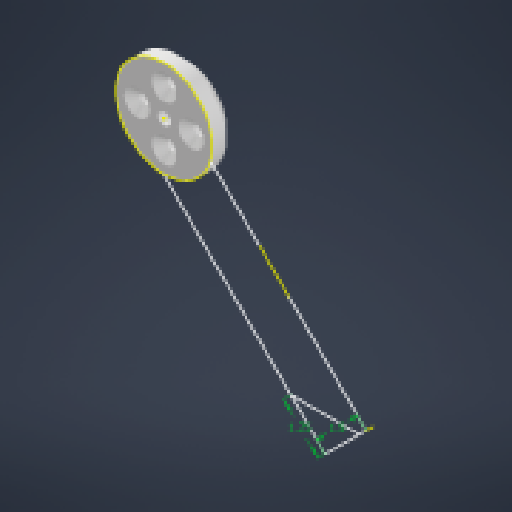
# Autodesk Inventor part: new_custom_servo_claw_bracket
Saved by Autodesk Inventor 2026 (Build 300175000, 175)
## iProperties
Created: 2025-03-29
Part Number: new_custom_servo_claw_bracket
Material: Generic
Document SubType Name: Modeling
Designer: paris
Density: 1 g/cm^3
Appearance: Default
Author: paris
Autodesk Inventor part; units mm, degrees
ref_plane "YZ Plane" through (0, 0, 0) normal (1, 0, 0) x (0, 1, 0)
ref_plane "XZ Plane" through (0, 0, 0) normal (0, 1, 0) x (-1, 0, 0)
ref_plane "XY Plane" through (0, 0, 0) normal (0, 0, 1) x (1, 0, 0)
sketch "Sketch1" plane through (0, 0, 0) normal (0, 0, 1) x (1, 0, 0)
  circle A0 centre (0, 0) radius 9.4
  circle A1 centre (4.949749, 4.949749) radius 1.25
  circle A2 centre (-4.949749, 4.949749) radius 1.25
  circle A3 centre (-4.949749, -4.949749) radius 1.25
  circle A4 centre (0, 0) radius 1.6
  circle A5 centre (4.949749, -4.949749) radius 1.25
  circle A6 centre (0, 0) radius 12.5
  circle A7 centre (0, 0) radius 3.75
  dimension "d0" = 25
  dimension "d31" = 7.5
  constraints: 2 centre point, 2 coincident
  measures "d0" diameter of A6
  measures "d31" diameter of A7
extrude "Extrusion1" add sketch "Sketch1" along normal blind 6 contours A0 | A6 | A7
sketch "Sketch3" plane through (0, 0, 0) normal (0, 1, 0) x (-1, 0, 0)
  line L0 (52.293085, -36.2) -> (52.293085, -39.2)
  line L1 (52.293085, -39.2) -> (35.480704, -39.2)
  line L2 (35.480704, -39.2) -> (35.480704, -35.2)
  line L3 (35.480704, -35.2) -> (51.293085, -35.2)
  line L4 (51.293085, -35.2) -> (52.293085, -36.2)
  line L5 (10.944606, 0.32) -> (11.944606, 1.32) construction
  line L6 (11.944606, 1.32) -> (38.508723, 1.32) construction
  line L7 (38.508723, 1.32) -> (39.508723, 0.32)
  line L8 (39.508723, 0.32) -> (39.508723, -1.18)
  line L9 (39.508723, -1.18) -> (10.944606, -1.18) construction
  line L10 (10.944606, -1.18) -> (10.944606, 0.32) construction
  line L11 (12.5, 0) -> (-12.5, 0)
  line L12 (12.5, 0) -> (10, 0)
  line L13 (12.5, 0) -> (12.5, 2.5)
  line L14 (12.5, 2.5) -> (10, 0)
  line L15 (0, -47.54) -> (0, 10.84)
  point P0 (0, 0)
  dimension "d9" = 2.5
  dimension "d10" = 2.5
  constraints: 28 end point, 4 horizontal, 4 vertical, 1 perpendicular, 1 point on line, 14 other
  measures "d9" distance of L11.start L12.end
  measures "d10" distance of L11.start L13.end
revolve "Revolution2" cut sketch "Sketch3" angle 360 about axis through (0, 0, -10) along (0, 0, 1) contours L11 L14 L13
sketch "Sketch4" plane through (0, 0, 6) normal (0, 0, 1) x (1, 0, 0)
  line L0 (24.631452, -16.169105) -> (32.233463, -23.771115)
  line L1 (24.631452, -16.169105) -> (11.991468, -3.529121)
  circle A0 centre (0, 0) radius 12.5
  line L2 (52.208369, -43.746021) -> (53.976136, -41.978255)
  line L3 (32.233463, -23.771115) -> (52.208369, -43.746021)
  line L4 (52.208369, -43.746021) -> (41.601767, -54.352623)
  line L5 (41.601767, -54.352623) -> (-12.497431, -0.253425)
  line L6 (50.440602, -45.513788) -> (32.762932, -45.513788)
  line L7 (11.991468, -3.529121) -> (10.223701, -1.761354)
  line L8 (10.223701, -1.761354) -> (-0.382901, -12.367955)
  line L9 (-0.382901, -12.367955) -> (-12.497431, -0.253425)
  point P0 (-0.382901, -12.367955)
  dimension "d12" = 15
  dimension "d13" = 12.5
  dimension "d20" = 2.5
  constraints: 16 end point, 3 collinear, 3 perpendicular, 2 point on circle, 2 point on line, 1 horizontal
  measures "d12" distance of L2.start L4.end
  measures "d13" distance of L4.end L6.end
  measures "d20" distance of L1.end L7.end
ref_plane "Work Plane1" through (-4.949749, -4.949749, 0) normal (-0.7071068, 0.7071068, 0) x (0, 0, 1)
extrude "Extrusion2" add sketch "Sketch4" against normal blind 6 contours L0 L3 L4 L6 L5 A0 L1 | A0 L5 L8 L7 picked at (4.096617, -8.795683)
sketch "Sketch5" plane through (-4.949749, -4.949749, 0) normal (-0.7071068, 0.7071068, 0) x (0, 0, 1)
  line L0 (0, -1.25) -> (6, -1.25)
  line L1 (6, -1.25) -> (6, -5.499998)
  line L2 (2.5, 19.500002) -> (6, 19.500002)
  line L3 (0, 17.000002) -> (2.5, 19.500002)
  line L4 (0, -2.999998) -> (0, -1.25)
  line L5 (6, 1.25) -> (0, 1.25)
  line L6 (0, 1.25) -> (0, 5.400002)
  line L7 (0, 5.400002) -> (6, 5.400002)
  line L8 (6, 5.400002) -> (6, 1.25)
  line L9 (6, 15.250004) -> (0, 15.250004)
  line L10 (6, 12.750004) -> (6, 8.600002)
  line L11 (6, 8.600002) -> (0, 8.600002)
  line L12 (0, 8.600002) -> (0, 12.750004)
  line L13 (0, 12.750004) -> (6, 12.750004)
  line L14 (2.5, -5.499998) -> (0, -2.999998)
  line L15 (6, -5.499998) -> (2.5, -5.499998)
  line L16 (6, -1.25) -> (4, -1.25)
  line L17 (6, -1.25) -> (6, -3.25)
  line L18 (6, 19.500002) -> (6, -5.499998)
  line L19 (6, -3.25) -> (4, -1.25)
  line L20 (-1.2, 0) -> (7.2, 0)
  line L21 (6, 19.500002) -> (6, 15.250004)
  line L22 (0, 15.250004) -> (0, 17.000002)
  point P0 (0, 7.000002)
  point P1 (6, -3.25)
  dimension "d14" = 2
  dimension "d15" = 2
  constraints: 6 end point, 1 point on line, 2 other
  measures "d14" distance of L0.end L16.end
  measures "d15" distance of L0.end L17.end
revolve "Revolution3" cut sketch "Sketch5" angle 360 about axis through (-4.949749, -4.949749, 0) along (0, 0, 1) contours L0 L1 L19
pattern_circular "Circular Pattern2" count 4 over 360 about axis through (0, 0, 0) along (0, 0, 1) of "Revolution3"
sketch "Sketch6" plane through (-0.382901, -12.367955, 2.373881) normal (-0.7071068, 0.7071068, 0) x (0.7071068, 0.7071068, 0)
  line L0 (15, 2.373881) -> (15, 1.999565)
  spline S0 degree 2 poles (15, 1.999565) (14.65611, 2.197917) (14.324628, 2.373881) knots 0 0 0 1 1 1 weights 1 1.00054985 1
  line L1 (14.324628, 2.373881) -> (15, 2.373881)
  line L2 (18.204755, -0.126119) -> (18.204755, -3.626119)
  line L3 (18.204755, -3.626119) -> (11.912374, -3.626119)
  line L4 (6.12006, -3.626119) -> (-0.172321, -3.626119)
  line L5 (-0.172321, -3.626119) -> (-0.172321, -0.126119)
  line L6 (0, 0) -> (0, 2.373881)
  line L7 (0, 2.373881) -> (3.707806, 2.373881)
  line L8 (3.707806, 2.373881) -> (14.324628, 2.373881)
  spline S1 degree 2 poles (3.707806, 2.373881) (2.050603, 1.49417) (0, 0) knots 0 0 0 1 1 1 weights 1 1.01402107 1
  point P0 (9.016217, 2.373881)
  constraints: 1 horizontal alignment, 4 other
extrude "Extrusion3" add sketch "Sketch6" along normal up to surface round surface about axis through (0, 0, 1.25) along (0, 0, -1) radius 11.25 half angle -45 far side no
sketch "Sketch7" plane through (50.440602, -45.513788, 0) normal (0.7071068, -0.7071068, 0) x (0.7071068, 0.7071068, 0)
  line L0 (-12.5, 6) -> (0, 6)
  line L1 (-12.5, 6) -> (-12.5, 0)
  line L2 (0, 0) -> (-12.5, 0)
  line L3 (0, 6) -> (0, 0)
  line L4 (0, 6) -> (2.5, 6)
  line L5 (0, 6) -> (0, 0)
  line L6 (2.5, 0) -> (0, 0)
  line L7 (2.5, 6) -> (2.5, 0)
  line L8 (-17.381295, 1.62) -> (-20.312925, 1.62)
  line L9 (-17.381295, 1.62) -> (-12.5, 1.62)
  line L10 (-12.5, 0) -> (-9.5, 0)
  line L11 (-9.5, 0) -> (-9.5, 2)
  line L12 (-9.5, 2) -> (-12.5, 2)
  line L13 (-12.5, 2) -> (-12.5, 0)
  line L14 (-9.5, 2) -> (-7.5, 0)
  line L15 (-9.5, 2) -> (-6.671573, 2) construction
  point P0 (-3.483783, 0)
  point P1 (-12.5, 2)
  dimension "d25" = 3
  dimension "d26" = 2
  dimension "d27" = 45
  constraints: 14 end point, 2 horizontal, 2 parallel, 2 perpendicular, 2 point on line, 1 equal length
  measures "d25" distance of L12.end L11.end
  measures "d26" distance of L11.end L10.end
  measures "d27" angle of L14 L15
extrude "Extrusion4" cut sketch "Sketch7" against normal up to surface contours L12 L11 L2 L1 | L14 L2 L11 round surface about axis through (0, 0, 1.25) along (0, 0, -1) radius 11.25 half angle -45 far side no
sketch "Sketch9" plane through (-4.949749, -4.949749, 0) normal (-0.7071068, 0.7071068, 0) x (0, 0, 1)
  line L0 (6, 17.250004) -> (4, 15.250004)
  line L1 (4, 15.250004) -> (0, 15.250004)
  line L2 (0, 15.250004) -> (0, 17.000002)
  line L3 (0, 17.000002) -> (2.5, 19.500002)
  line L4 (2.5, 19.500002) -> (6, 19.500002)
  line L5 (6, 19.500002) -> (6, 17.250004)
  line L6 (4, 12.750004) -> (6, 10.750004)
  line L7 (6, 10.750004) -> (6, 8.600002)
  line L8 (6, 8.600002) -> (0, 8.600002)
  line L9 (0, 8.600002) -> (0, 12.750004)
  line L10 (0, 12.750004) -> (4, 12.750004)
  line L11 (4, -1.25) -> (6, -3.25)
  line L12 (6, -3.25) -> (6, -5.499998)
  line L13 (6, -5.499998) -> (2.5, -5.499998)
  line L14 (2.5, -5.499998) -> (0, -2.999998)
  line L15 (0, -2.999998) -> (0, -1.25)
  line L16 (0, -1.25) -> (4, -1.25)
  line L17 (6, 3.25) -> (4, 1.25)
  line L18 (4, 1.25) -> (0, 1.25)
  line L19 (0, 1.25) -> (0, 5.400002)
  line L20 (0, 5.400002) -> (6, 5.400002)
  line L21 (6, 5.400002) -> (6, 3.25)
  line L22 (2.5, -5.499998) -> (2.5, 19.500002)
  line L23 (6, 12.983785) -> (2.5, 12.983785)
  line L24 (2.5, 12.983785) -> (2.5, -2.016215)
  line L25 (2.5, -2.016215) -> (6, -2.016215)
  line L26 (6, 12.983785) -> (6, -2.016215)
  line L27 (0, 8.600002) -> (0, 5.400002)
  line L28 (0, 5.400002) -> (0, 8.600002)
  line L29 (0, 7.000002) -> (2.5, 7.000002)
  line L30 (2.5, 7.000002) -> (2.5, 11.000002)
  line L31 (2.5, 11.000002) -> (0, 11.000002)
  line L32 (2.5, 7.000002) -> (2.5, 3.000002)
  line L33 (2.5, 3.000002) -> (0, 2.983785)
  point P0 (2.5, 11.000002)
  dimension "d32" = 2.5
  dimension "d33" = 4
  dimension "d34" = 4
  constraints: 12 end point, 3 perpendicular, 3 point on line
  measures "d32" distance of L29.start L29.end
  measures "d33" distance of L29.end L30.end
  measures "d34" distance of L29.end L32.end
extrude "Extrusion5" cut sketch "Sketch9" along normal blind 25 contours L22 L8 L9 L31 | L22 L29 L27 L8 | L22 L20 L27 L29 | L22 L33 L19 L20
sketch "Sketch10" plane through (-4.949749, -4.949749, 0) normal (-0.7071068, 0.7071068, 0) x (-0.7071068, -0.7071068, 0)
  line L0 (-8.600002, 2.5) -> (-8.600002, 0)
  line L1 (-8.600002, 2.5) -> (-11.000002, 2.5)
  line L2 (-11.000002, 2.5) -> (-11.000002, 0)
  line L3 (-8.600002, 0) -> (-11.000002, 0)
  line L4 (-7.000002, -1.2) -> (-7.000002, 7.2)
  point P0 (-7.000002, 0)
revolve "Revolution4" cut sketch "Sketch10" angle 360 about axis through (0, 0, -10) along (0, 0, 1)
ref_plane "Work Plane2" through (0, 0, -18.75) normal (0, 0, -1) x (-1, 0, 0)
mirror "Mirror1" about plane through (0, 0, -18.75) normal (0, 0, -1) of "Extrusion4", "Extrusion3", "Revolution3", "Circular Pattern2", "Extrusion2", "Revolution2", "Extrusion1"
sketch "Sketch11" plane through (52.208369, -43.746021, 6) normal (0.7071068, 0.7071068, 0) x (0, 0, -1)
  arc A0 (36.443783, 18.378448) -> (35.045362, 17.55589) centre (36.443783, 16.778448) ccw
  arc A1 (33.809543, 17.615975) -> (35.045362, 17.55589) centre (34.442292, 17.891162) ccw
  arc A2 (33.809543, 17.615975) -> (30.083918, 17.860337) centre (31.883783, 16.778448) ccw
  arc A3 (28.824133, 18.044523) -> (30.083918, 17.860337) centre (29.492533, 18.215815) ccw
  arc A4 (28.824133, 18.044523) -> (18.943434, 18.044523) centre (23.883783, 16.778448) ccw
  arc A5 (17.683649, 17.860337) -> (18.943434, 18.044523) centre (18.275033, 18.215815) ccw
  arc A6 (17.683649, 17.860337) -> (13.958024, 17.615975) centre (15.883783, 16.778448) ccw
  arc A7 (12.722205, 17.55589) -> (13.958024, 17.615975) centre (13.325275, 17.891162) ccw
  arc A8 (12.722205, 17.55589) -> (11.323783, 18.378448) centre (11.323783, 16.778448) ccw
  line L0 (11.323783, 22.635) -> (11.323783, 18.378448)
  line L1 (5.71, 28.248783) -> (11.323783, 22.635)
  line L2 (5.71, 38.99965) -> (5.71, 28.248783)
  arc A9 (5.71, 38.99965) -> (6.096638, 39.441716) centre (5.183783, 39.85) ccw
  arc A10 (6.726508, 39.85) -> (6.096638, 39.441716) centre (6.726508, 39.16) ccw
  line L3 (7.800239, 39.85) -> (6.726508, 39.85)
  arc A11 (7.800239, 39.85) -> (8.252787, 40.037452) centre (7.800239, 40.49) ccw
  line L4 (11.21157, 42.996234) -> (8.252787, 40.037452)
  arc A12 (12.296639, 42.446127) -> (11.21157, 42.996234) centre (11.664118, 42.543686) ccw
  arc A13 (12.296639, 42.446127) -> (14.459982, 42.506034) centre (13.383783, 42.278448) ccw
  arc A14 (15.086135, 43.278448) -> (14.459982, 42.506034) centre (15.086135, 42.638448) ccw
  line L5 (15.853783, 43.278448) -> (15.086135, 43.278448)
  arc A15 (16.493783, 42.638448) -> (15.853783, 43.278448) centre (15.853783, 42.638448) ccw
  line L6 (16.493783, 42.638448) -> (16.493783, 27.277734)
  arc A16 (16.493783, 27.277734) -> (18.393783, 25.377734) centre (18.393783, 27.277734) ccw
  line L7 (18.393783, 25.377734) -> (29.373783, 25.377734)
  arc A17 (29.373783, 25.377734) -> (31.273783, 27.277734) centre (29.373783, 27.277734) ccw
  line L8 (31.273783, 27.277734) -> (31.273783, 42.638448)
  arc A18 (31.913783, 43.278448) -> (31.273783, 42.638448) centre (31.913783, 42.638448) ccw
  line L9 (32.681432, 43.278448) -> (31.913783, 43.278448)
  arc A19 (33.307584, 42.506034) -> (32.681432, 43.278448) centre (32.681432, 42.638448) ccw
  arc A20 (33.307584, 42.506034) -> (35.470928, 42.446127) centre (34.383783, 42.278448) ccw
  arc A21 (36.555997, 42.996234) -> (35.470928, 42.446127) centre (36.103449, 42.543686) ccw
  line L10 (39.51478, 40.037452) -> (36.555997, 42.996234)
  arc A22 (39.51478, 40.037452) -> (39.967328, 39.85) centre (39.967328, 40.49) ccw
  line L11 (41.041059, 39.85) -> (39.967328, 39.85)
  arc A23 (41.670929, 39.441716) -> (41.041059, 39.85) centre (41.041059, 39.16) ccw
  arc A24 (41.670929, 39.441716) -> (42.057567, 38.99965) centre (42.583783, 39.85) ccw
  line L12 (42.057567, 28.248783) -> (42.057567, 38.99965)
  line L13 (36.443783, 22.635) -> (42.057567, 28.248783)
  line L14 (36.443783, 18.378448) -> (36.443783, 22.635)
  circle A25 centre (36.443783, 36.16) radius 1.6
  circle A26 centre (11.323783, 36.16) radius 1.6
  circle A27 centre (13.383783, 28.778448) radius 1.1
  circle A28 centre (34.383783, 28.778448) radius 1.1
  arc A29 (35.045362, 16.001006) -> (36.443783, 15.178448) centre (36.443783, 16.778448) ccw
  line L15 (36.443783, 9.11) -> (36.443783, 15.178448)
  line L16 (28.414559, 1.080776) -> (36.443783, 9.11)
  arc A30 (25.805335, 0) -> (28.414559, 1.080776) centre (25.805335, 3.69) ccw
  line L17 (21.962231, 0) -> (25.805335, 0)
  arc A31 (19.353007, 1.080776) -> (21.962231, 0) centre (21.962231, 3.69) ccw
  line L18 (11.323783, 9.11) -> (19.353007, 1.080776)
  line L19 (11.323783, 15.178448) -> (11.323783, 9.11)
  arc A32 (11.323783, 15.178448) -> (12.722205, 16.001006) centre (11.323783, 16.778448) ccw
  arc A33 (13.958024, 15.940921) -> (12.722205, 16.001006) centre (13.325275, 15.665734) ccw
  arc A34 (13.958024, 15.940921) -> (17.683649, 15.696559) centre (15.883783, 16.778448) ccw
  arc A35 (18.943434, 15.512374) -> (17.683649, 15.696559) centre (18.275033, 15.341081) ccw
  arc A36 (18.943434, 15.512374) -> (22.617709, 11.838098) centre (23.883783, 16.778448) ccw
  arc A37 (22.801894, 10.578314) -> (22.617709, 11.838098) centre (22.446417, 11.169698) ccw
  arc A38 (22.801894, 10.578314) -> (24.965672, 10.578314) centre (23.883783, 8.778448) ccw
  arc A39 (25.149858, 11.838098) -> (24.965672, 10.578314) centre (25.32115, 11.169698) ccw
  arc A40 (25.149858, 11.838098) -> (28.824133, 15.512374) centre (23.883783, 16.778448) ccw
  arc A41 (30.083918, 15.696559) -> (28.824133, 15.512374) centre (29.492533, 15.341081) ccw
  arc A42 (30.083918, 15.696559) -> (33.809543, 15.940921) centre (31.883783, 16.778448) ccw
  arc A43 (35.045362, 16.001006) -> (33.809543, 15.940921) centre (34.442292, 15.665734) ccw
  circle A44 centre (23.883783, 3.69) radius 1.6
  line L20 (16.493783, 42.638448) -> (31.273783, 42.638448)
  line L21 (6, 0) -> (6, 59.837863)
  line L22 (43.5, 58.691943) -> (43.5, 7.5)
  line L23 (6, 0) -> (43.5, 0)
  line L24 (43.5, 0) -> (43.5, 45)
  line L25 (43.5, 45) -> (6, 45)
  line L26 (6, 45) -> (6, 0)
  line L27 (13.5, 45) -> (6, 52.5)
  line L28 (13.5, 45) -> (24.106602, 45) construction
  line L29 (36, 45) -> (43.5, 52.5)
  line L30 (36, 45) -> (46.606602, 45) construction
  line L31 (11.323783, 15.178448) -> (11.323783, 18.378448)
  line L32 (36.443783, 18.378448) -> (36.443783, 15.178448)
  line L33 (10.823783, 15.178448) -> (10.823783, 18.378448)
  arc A45 (34.608355, 15.758055) -> (36.443783, 14.678448) centre (36.443783, 16.778448) ccw
  arc A46 (34.608355, 15.758055) -> (34.268057, 15.74151) centre (34.442292, 15.665734) ccw
  arc A47 (29.655378, 15.438967) -> (34.268057, 15.74151) centre (31.883783, 16.778448) ccw
  arc A48 (29.655378, 15.438967) -> (29.308481, 15.388249) centre (29.492533, 15.341081) ccw
  arc A49 (25.273983, 11.35375) -> (29.308481, 15.388249) centre (23.883783, 16.778448) ccw
  arc A50 (25.273983, 11.35375) -> (25.223265, 11.006853) centre (25.32115, 11.169698) ccw
  arc A51 (22.544302, 11.006853) -> (25.223265, 11.006853) centre (23.883783, 8.778448) ccw
  arc A52 (22.544302, 11.006853) -> (22.493584, 11.35375) centre (22.446417, 11.169698) ccw
  arc A53 (18.459086, 15.388249) -> (22.493584, 11.35375) centre (23.883783, 16.778448) ccw
  arc A54 (18.459086, 15.388249) -> (18.112188, 15.438967) centre (18.275033, 15.341081) ccw
  arc A55 (13.49951, 15.74151) -> (18.112188, 15.438967) centre (15.883783, 16.778448) ccw
  arc A56 (13.49951, 15.74151) -> (13.159212, 15.758055) centre (13.325275, 15.665734) ccw
  arc A57 (11.323783, 14.678448) -> (13.159212, 15.758055) centre (11.323783, 16.778448) ccw
  arc A58 (13.159212, 17.798841) -> (11.323783, 18.878448) centre (11.323783, 16.778448) ccw
  arc A59 (13.159212, 17.798841) -> (13.49951, 17.815386) centre (13.325275, 17.891162) ccw
  arc A60 (18.112188, 18.11793) -> (13.49951, 17.815386) centre (15.883783, 16.778448) ccw
  arc A61 (18.112188, 18.11793) -> (18.459086, 18.168648) centre (18.275033, 18.215815) ccw
  arc A62 (29.308481, 18.168648) -> (18.459086, 18.168648) centre (23.883783, 16.778448) ccw
  arc A63 (29.308481, 18.168648) -> (29.655378, 18.11793) centre (29.492533, 18.215815) ccw
  arc A64 (34.268057, 17.815386) -> (29.655378, 18.11793) centre (31.883783, 16.778448) ccw
  arc A65 (34.268057, 17.815386) -> (34.608355, 17.798841) centre (34.442292, 17.891162) ccw
  arc A66 (36.443783, 18.878448) -> (34.608355, 17.798841) centre (36.443783, 16.778448) ccw
  line L34 (36.943783, 18.378448) -> (36.943783, 15.178448)
  circle A67 centre (23.883783, 3.69) radius 2.1
  line L35 (31.773783, 42.638448) -> (31.773783, 27.277734)
  arc A68 (29.373783, 24.877734) -> (31.773783, 27.277734) centre (29.373783, 27.277734) ccw
  line L36 (29.373783, 24.877734) -> (18.393783, 24.877734)
  arc A69 (15.993783, 27.277734) -> (18.393783, 24.877734) centre (18.393783, 27.277734) ccw
  line L37 (15.993783, 27.277734) -> (15.993783, 42.638448)
  line L38 (16.493783, 43.138448) -> (31.273783, 43.138448)
  line L39 (16.493783, 43.138448) -> (15.993783, 42.638448)
  line L40 (31.273783, 43.138448) -> (31.773783, 42.638448)
  line L41 (11.323783, 18.878448) -> (10.823783, 18.378448)
  line L42 (10.823783, 15.178448) -> (11.323783, 14.678448)
  line L43 (36.443783, 18.878448) -> (36.943783, 18.378448)
  line L44 (36.943783, 15.178448) -> (36.443783, 14.678448)
  point P0 (6, 67.85)
  point P1 (25.805335, 0)
  point P2 (6, 45)
  dimension "d38" = 45
  dimension "d39" = 135
  dimension "d40" = 45
  dimension "d41" = 7.5
  dimension "d42" = 7.5
  dimension "d43" = 0.5
  dimension "d44" = 0.5
  dimension "d45" = 0.5
  dimension "d46" = 0.5
  dimension "d47" = 0.5
  dimension "d48" = 0.5
  dimension "d49" = 0.5
  constraints: 48 point on circle, 40 end point, 25 centre point, 6 parallel, 5 perpendicular, 5 point on line, 3 horizontal, 2 equal length, 24 other
  measures "d38" distance of L24.end L23.end
  measures "d39" angle of L28 L27
  measures "d40" angle of L30 L29
  measures "d41" distance of L24.end L29.end
  measures "d42" distance of L25.end L27.end
  measures "d43" distance between parallel lines of L31 L33
  measures "d44" radial gap between concentric circles of A34 A55
  measures "d45" radial gap between concentric circles of A4 A62
  measures "d46" distance between parallel lines of L32 L34
  measures "d47" radial gap between concentric circles of A44 A67
  measures "d48" distance between parallel lines of L7 L36
  measures "d49" distance between parallel lines of L20 L38
extrude "Extrusion6" add sketch "Sketch11" against normal blind 3.5 contours A66 A65 A64 A63 A62 A61 A60 A59 A58 L0 L1 L21 A9 A10 L3 A11 L4 A12 A13 A14 L5 A15 L39 L37 A69 L36 A68 L35 L40 A18 L9 A19 A20 A21 L10 A22 L11 A23 A24 L12 L13 L14 | L14 L13 L12 A24 A23 L11 A22 L10 A21 A20 A19 L9 A18 L40 L38 L39 A15 L5 A14 A13 A12 L4 A11 L3 A10 A9 L21 L25 L22 L24 L23 A30 L16 L15 L44 L34 L43 | L15 L16 A30 L17 A31 L18 L19 A57 A56 A55 A54 A53 A52 A51 A50 A49 A48 A47 A46 A45 | L23 L21 L1 L0 L41 L33 L42 L19 L18 A31 | L25 L29 L22 | L21 L27 L25 | A25 | A26 | A27 | A28
sketch "Sketch12" plane through (49.733495, -46.220895, 6) normal (-0.7071068, -0.7071068, 0) x (0, 0, 1)
  line L0 (-43.5, 0) -> (-6, 0)
  line L1 (-6, 0) -> (-6, 1)
  line L2 (-6, 52.5) -> (-6, 1)
  line L3 (-6, 52.5) -> (-13.5, 45)
  line L4 (-13.5, 45) -> (-36, 45)
  line L5 (-36, 45) -> (-43.5, 52.5)
  line L6 (-43.5, 1) -> (-43.5, 52.5)
  line L7 (-43.5, 1) -> (-43.5, 0)
  line L8 (-31.773783, 42.638448) -> (-31.273783, 43.138448)
  line L9 (-31.273783, 43.138448) -> (-16.493783, 43.138448)
  line L10 (-16.493783, 43.138448) -> (-15.993783, 42.638448)
  line L11 (-15.993783, 42.638448) -> (-15.993783, 27.277734)
  arc A0 (-18.393783, 24.877734) -> (-15.993783, 27.277734) centre (-18.393783, 27.277734) ccw
  line L12 (-18.393783, 24.877734) -> (-29.373783, 24.877734)
  arc A1 (-31.773783, 27.277734) -> (-29.373783, 24.877734) centre (-29.373783, 27.277734) ccw
  line L13 (-31.773783, 27.277734) -> (-31.773783, 42.638448)
  circle A2 centre (-23.883783, 3.69) radius 2.1
  line L14 (-36.943783, 18.378448) -> (-36.443783, 18.878448)
  arc A3 (-34.608355, 17.798841) -> (-36.443783, 18.878448) centre (-36.443783, 16.778448) ccw
  arc A4 (-34.608355, 17.798841) -> (-34.268057, 17.815386) centre (-34.442292, 17.891162) ccw
  arc A5 (-29.655378, 18.11793) -> (-34.268057, 17.815386) centre (-31.883783, 16.778448) ccw
  arc A6 (-29.655378, 18.11793) -> (-29.308481, 18.168648) centre (-29.492533, 18.215815) ccw
  arc A7 (-18.459086, 18.168648) -> (-29.308481, 18.168648) centre (-23.883783, 16.778448) ccw
  arc A8 (-18.459086, 18.168648) -> (-18.112188, 18.11793) centre (-18.275033, 18.215815) ccw
  arc A9 (-13.49951, 17.815386) -> (-18.112188, 18.11793) centre (-15.883783, 16.778448) ccw
  arc A10 (-13.49951, 17.815386) -> (-13.159212, 17.798841) centre (-13.325275, 17.891162) ccw
  arc A11 (-11.323783, 18.878448) -> (-13.159212, 17.798841) centre (-11.323783, 16.778448) ccw
  line L15 (-11.323783, 18.878448) -> (-10.823783, 18.378448)
  line L16 (-10.823783, 18.378448) -> (-10.823783, 15.178448)
  line L17 (-10.823783, 15.178448) -> (-11.323783, 14.678448)
  arc A12 (-13.159212, 15.758055) -> (-11.323783, 14.678448) centre (-11.323783, 16.778448) ccw
  arc A13 (-13.159212, 15.758055) -> (-13.49951, 15.74151) centre (-13.325275, 15.665734) ccw
  arc A14 (-18.112188, 15.438967) -> (-13.49951, 15.74151) centre (-15.883783, 16.778448) ccw
  arc A15 (-18.112188, 15.438967) -> (-18.459086, 15.388249) centre (-18.275033, 15.341081) ccw
  arc A16 (-22.493584, 11.35375) -> (-18.459086, 15.388249) centre (-23.883783, 16.778448) ccw
  arc A17 (-22.493584, 11.35375) -> (-22.544302, 11.006853) centre (-22.446417, 11.169698) ccw
  arc A18 (-25.223265, 11.006853) -> (-22.544302, 11.006853) centre (-23.883783, 8.778448) ccw
  arc A19 (-25.223265, 11.006853) -> (-25.273983, 11.35375) centre (-25.32115, 11.169698) ccw
  arc A20 (-29.308481, 15.388249) -> (-25.273983, 11.35375) centre (-23.883783, 16.778448) ccw
  arc A21 (-29.308481, 15.388249) -> (-29.655378, 15.438967) centre (-29.492533, 15.341081) ccw
  arc A22 (-34.268057, 15.74151) -> (-29.655378, 15.438967) centre (-31.883783, 16.778448) ccw
  arc A23 (-34.268057, 15.74151) -> (-34.608355, 15.758055) centre (-34.442292, 15.665734) ccw
  arc A24 (-36.443783, 14.678448) -> (-34.608355, 15.758055) centre (-36.443783, 16.778448) ccw
  line L18 (-36.443783, 14.678448) -> (-36.943783, 15.178448)
  line L19 (-36.943783, 15.178448) -> (-36.943783, 18.378448)
  point P0 (-6, 67.85)
extrude "Extrusion7" add sketch "Sketch12" along normal blind 3.5 contours L7 L6 L5 L4 L3 L2 L1 L0 | L8 L9 L10 L11 A0 L12 A1 L13 | A2 | L14 A3 A4 A5 A6 A7 A8 A9 A10 A11 L15 L16 L17 A12 A13 A14 A15 A16 A17 A18 A19 A20 A21 A22 A23 A24 L18 L19
sketch "Sketch13" plane through (44.076641, -45.513788, 0) normal (0, 0, 1) x (1, 0, 0)
  line L0 (6.363961, 0) -> (0, 0)
  line L1 (3.181981, -3.181981) -> (0, 0)
  line L2 (6.363961, 0) -> (3.181981, -3.181981)
  point P0 (-44.076641, 45.513788)
extrude "Extrusion8" cut sketch "Sketch13" against normal through all
sketch "Sketch14" plane through (-0.253425, -12.497431, 2.5) normal (-0.7071068, -0.7071068, 0) x (0, 0, 1)
  line L0 (3.5, -59.192181) -> (-46, -59.192181)
  line L1 (3.5, -46.692181) -> (3.5, -59.192181)
  line L2 (3.5, 0) -> (3.5, -46.692181)
  line L3 (-46, 0) -> (-46, -46.692181)
  line L4 (-46, -46.692181) -> (-46, -59.192181)
  line L5 (-2.21, -20.192531) -> (-2.21, -30.943397) construction
  line L6 (-2.21, -30.943397) -> (-7.823783, -36.557181) construction
  line L7 (-7.823783, -36.557181) -> (-7.823783, -40.813733) construction
  line L8 (-7.823783, -44.013733) -> (-7.823783, -50.082181) construction
  line L9 (-7.823783, -50.082181) -> (-15.853007, -58.111405)
  arc A0 (-18.462231, -59.192181) -> (-15.853007, -58.111405) centre (-18.462231, -55.502181) ccw
  line L10 (-7.823783, -40.813733) -> (-7.823783, -44.013733) construction
  line L11 (-2.21, -20.192531) -> (3.5, -14.482531) construction
  line L12 (-2.21, -20.192531) -> (5.865159, -20.192531) construction
  line L13 (3.5, -19.702914) -> (-0.5, -23.702914)
  line L14 (-0.5, 0.738991) -> (-0.5, -46.692181)
  line L15 (3.5, -19.702914) -> (9.156854, -19.702914) construction
  line L16 (-0.5, -23.702914) -> (-0.5, -33.702914)
  line L17 (-0.5, -33.702914) -> (-4.035534, -37.238448)
  line L18 (-7.823783, -50.082181) -> (-4.035534, -46.293931)
  line L19 (-4.035534, -46.293931) -> (-4.035534, -37.238448)
  line L20 (-21.25, -59.192181) -> (-21.25, -14.192181)
  line L21 (-32.5, -14.192181) -> (-10, -14.192181)
  line L22 (-34.676217, -50.082181) -> (-26.646993, -58.111405)
  arc A1 (-26.646993, -58.111405) -> (-24.037769, -59.192181) centre (-24.037769, -55.502181) ccw
  line L23 (-46, -19.702914) -> (-42, -23.702914)
  line L24 (-42, -23.702914) -> (-42, -33.702914)
  line L25 (-42, -33.702914) -> (-38.464466, -37.238448)
  line L26 (-34.676217, -50.082181) -> (-38.464466, -46.293931)
  line L27 (-38.464466, -46.293931) -> (-38.464466, -37.238448)
  point P0 (-2.5, 8.657819)
  point P1 (-24.037769, -59.192181)
  dimension "d56" = 45
  dimension "d57" = 135
  dimension "d58" = 10
  dimension "d59" = 5
  dimension "d60" = 135
  constraints: 32 end point, 9 symmetric about line, 4 point on line, 2 equal length, 2 horizontal, 2 midpoint, 2 point on circle, 2 vertical, 1 centre point, 1 parallel, 1 other
  measures "d56" angle of L12 L11
  measures "d57" angle of L13 L15
  measures "d58" distance of L13.end L16.end
  measures "d59" distance of L16.end L17.end
  measures "d60" angle of L16 L17
extrude "Extrusion9" cut sketch "Sketch14" against normal through all
equation "\"d35\" = d0"
body "Solid1"
